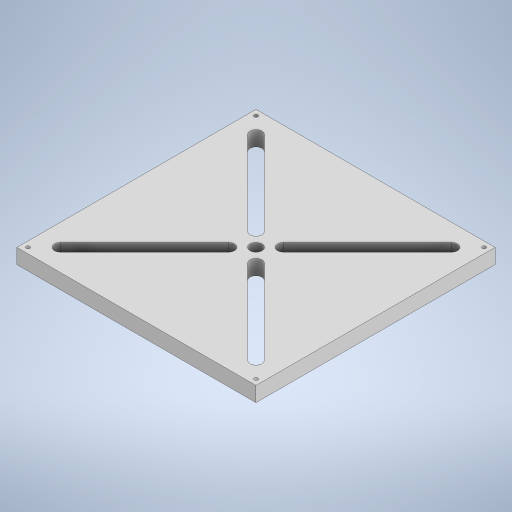
# Autodesk Inventor part: Layer 5
Saved by Autodesk Inventor 2023 (Build 270158000, 158)
## iProperties
Created: 2023-04-21
Part Number: Layer 5
Material: Generic
Document SubType Name: Modeling
Designer: byrne
Density: 1 g/cm^3
Appearance: Default
Author: byrne
Autodesk Inventor part; units mm, degrees
ref_plane "YZ Plane" through (0, 0, 0) normal (1, 0, 0) x (0, 1, 0)
ref_plane "XZ Plane" through (0, 0, 0) normal (0, 1, 0) x (-1, 0, 0)
ref_plane "XY Plane" through (0, 0, 0) normal (0, 0, 1) x (1, 0, 0)
sketch "Sketch1" plane through (0, 0, 0) normal (0, 1, 0) x (-1, 0, 0)
  line L0 (0, 0) -> (101.6, 0)
  line L1 (101.6, 0) -> (101.6, -101.6)
  line L2 (101.6, -101.6) -> (0, -101.6)
  line L3 (0, -101.6) -> (0, 0)
  line L4 (4.7625, -96.8375) -> (96.8375, -96.8375)
  line L5 (96.8375, -96.8375) -> (96.8375, -4.7625)
  line L6 (96.8375, -4.7625) -> (4.7625, -4.7625)
  line L7 (4.7625, -4.7625) -> (4.7625, -96.8375)
  line L8 (96.8375, -4.7625) -> (4.7625, -96.8375) construction
  circle A0 centre (50.8, -50.8) radius 2.5527
  circle A1 centre (50.8, -50.8) radius 5.7277
  line L9 (54.850096, -46.749904) -> (94.143423, -7.456577) construction
  line L10 (58.442198, -46.749904) -> (94.143423, -11.048679)
  line L11 (90.551321, -7.456577) -> (54.850096, -43.157802)
  arc A2 (54.850096, -43.157802) -> (58.442198, -46.749904) centre (56.646147, -44.953853) ccw
  arc A3 (94.143423, -11.048679) -> (90.551321, -7.456577) centre (92.347372, -9.252628) ccw
  line L12 (46.749904, -43.157802) -> (11.048679, -7.456577)
  arc A4 (43.157802, -46.749904) -> (46.749904, -43.157802) centre (44.953853, -44.953853) ccw
  line L13 (7.456577, -11.048679) -> (43.157802, -46.749904)
  arc A5 (11.048679, -7.456577) -> (7.456577, -11.048679) centre (9.252628, -9.252628) ccw
  line L14 (43.157802, -54.850096) -> (7.456577, -90.551321)
  arc A6 (46.749904, -58.442198) -> (43.157802, -54.850096) centre (44.953853, -56.646147) ccw
  line L15 (11.048679, -94.143423) -> (46.749904, -58.442198)
  arc A7 (7.456577, -90.551321) -> (11.048679, -94.143423) centre (9.252628, -92.347372) ccw
  line L16 (54.850096, -58.442198) -> (90.551321, -94.143423)
  arc A8 (58.442198, -54.850096) -> (54.850096, -58.442198) centre (56.646147, -56.646147) ccw
  line L17 (94.143423, -90.551321) -> (58.442198, -54.850096)
  arc A9 (90.551321, -94.143423) -> (94.143423, -90.551321) centre (92.347372, -92.347372) ccw
  point P0 (0, -50.8)
  point P1 (74.496759, -27.103241)
  dimension "d0" = 101.6
  dimension "d1" = 101.6
  dimension "d2" = 4.7625
  dimension "d33" = 5.1054
  dimension "d34" = 3.175
  dimension "d35" = 5.08
  dimension "d36" = 6.35
  dimension "d39" = 360
  constraints: 38 end point, 18 point on circle, 9 centre point, 5 parallel, 4 point on line, 4 tangent, 3 midpoint, 2 perpendicular, 1 horizontal, 47 other
  measures "d0" distance of L1.end L2.end
  measures "d1" distance of L0.end L1.end
  measures "d2" distance between parallel lines of L2 L4
  measures "d33" diameter of A0
  measures "d35" diameter of A3
  measures "d36" distance of L5.end A3.centre
extrude "Extrusion1" add sketch "Sketch1" along normal blind 6.35 contours L0 L1 L2 L3 | L7 L6 L5 L4 | A1
sketch "Sketch2" plane through (0, 6.35, 0) normal (0, 1, 0) x (1, 0, 0)
  line L0 (0, 101.6) -> (-101.6, 101.6)
  line L1 (-101.6, 101.6) -> (-101.6, 0)
  line L2 (-101.6, 0) -> (0, 0)
  line L3 (0, 0) -> (0, 101.6)
  circle A0 centre (-99.21875, 99.21875) radius 0.79375
  circle A1 centre (-99.21875, 2.38125) radius 0.79375
  circle A2 centre (-2.38125, 99.21875) radius 0.79375
  circle A3 centre (-2.38125, 2.38125) radius 0.79375
  dimension "d20" = 1.5875
  dimension "d21" = 2.38125
  dimension "d22" = 2.38125
  dimension "d25" = 96.8375
  dimension "d28" = 96.8375
  constraints: 4 centre point, 1 horizontal, 1 vertical, 6 other
  measures "d20" diameter of A0
  measures "d21" distance from line of L0 A0.centre
  measures "d22" distance from line of L1 A0.centre
  measures "d25" distance of A0.centre A1.centre
  measures "d28" distance of A0.centre A2.centre
extrude "Extrusion2" cut sketch "Sketch2" against normal blind 6.35 contours A0 | A1 | A2 | A3
sketch "Sketch3" plane through (0, 6.35, 0) normal (0, 1, 0) x (1, 0, 0)
  circle A0 centre (-99.21875, 99.21875) radius 0.79375
  circle A1 centre (-99.21875, 2.38125) radius 0.79375
  circle A2 centre (-2.38125, 99.21875) radius 0.79375
  circle A3 centre (-2.38125, 2.38125) radius 0.79375
  line L0 (0, 101.6) -> (-101.6, 101.6)
  line L1 (-101.6, 101.6) -> (-101.6, 0)
  line L2 (-101.6, 0) -> (0, 0)
  line L3 (0, 0) -> (0, 101.6)
  arc A4 (-58.442198, 54.850096) -> (-54.850096, 58.442198) centre (-56.646147, 56.646147) ccw
  line L4 (-58.442198, 54.850096) -> (-94.143423, 90.551321)
  arc A5 (-90.551321, 94.143423) -> (-94.143423, 90.551321) centre (-92.347372, 92.347372) ccw
  line L5 (-90.551321, 94.143423) -> (-54.850096, 58.442198)
  circle A6 centre (-50.8, 50.8) radius 2.5527
  arc A7 (-46.749904, 58.442198) -> (-43.157802, 54.850096) centre (-44.953853, 56.646147) ccw
  line L6 (-46.749904, 58.442198) -> (-11.048679, 94.143423)
  arc A8 (-7.456577, 90.551321) -> (-11.048679, 94.143423) centre (-9.252628, 92.347372) ccw
  line L7 (-7.456577, 90.551321) -> (-43.157802, 54.850096)
  arc A9 (-43.157802, 46.749904) -> (-46.749904, 43.157802) centre (-44.953853, 44.953853) ccw
  line L8 (-43.157802, 46.749904) -> (-7.456577, 11.048679)
  arc A10 (-11.048679, 7.456577) -> (-7.456577, 11.048679) centre (-9.252628, 9.252628) ccw
  line L9 (-11.048679, 7.456577) -> (-46.749904, 43.157802)
  arc A11 (-54.850096, 43.157802) -> (-58.442198, 46.749904) centre (-56.646147, 44.953853) ccw
  line L10 (-54.850096, 43.157802) -> (-90.551321, 7.456577)
  arc A12 (-94.143423, 11.048679) -> (-90.551321, 7.456577) centre (-92.347372, 9.252628) ccw
  line L11 (-94.143423, 11.048679) -> (-58.442198, 46.749904)
body "Solid1"
